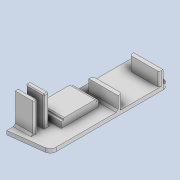
# Autodesk Inventor part: ploh
Saved by Autodesk Inventor 2020 (Build 240168000, 168)
## iProperties
Created: 2022-02-12
Part Number: ploh
Material: Типовые
Document SubType Name: Modeling
Designer: korra
Density: 1 g/cm^3
Appearance: По умолчанию
Author: korra
Autodesk Inventor part; units mm, degrees
ref_plane "YZ Plane" through (0, 0, 0) normal (1, 0, 0) x (0, 1, 0)
ref_plane "XZ Plane" through (0, 0, 0) normal (0, 1, 0) x (-1, 0, 0)
ref_plane "XY Plane" through (0, 0, 0) normal (0, 0, 1) x (1, 0, 0)
sketch "Эскиз1" plane through (0, 0, 0) normal (0, 1, 0) x (-1, 0, 0)
  line L0 (-5, 11.7093) -> (-5, -48.2907)
  line L1 (15, 10.2093) -> (15, -46.7907)
  line L2 (15, 10.2093) -> (15, 14.2093)
  line L3 (15, -46.7907) -> (15, -50.7907)
  line L4 (15, 14.2093) -> (-5, 11.7093)
  line L5 (15, -50.7907) -> (-5, -48.2907)
  point P0 (0, 0)
  dimension "d0" = 60
  dimension "d3" = 20
  dimension "d4" = 4
  dimension "d5" = 4
  constraints: 12 end point, 4 vertical
  measures "d0" distance of L0.start L0.end
  measures "d3" distance between parallel lines of L0 L1
  measures "d4" distance of L1.start L2.end
  measures "d5" distance of L1.end L3.end
extrude "Выдавливание1" add sketch "Эскиз1" along normal blind 2
fillet "Сопряжение1" radius 3 2 edges at (5, 1, -48.2907) (5, 1, 11.7093)
sketch "Эскиз3" plane through (0, 2, 0) normal (0, 1, 0) x (1, 0, 0)
  arc A0 (5, 45.6424) -> (2.3721, 48.6192) centre (2, 45.6424) ccw projected
  line L0 (5, 45.6424) -> (-10, 45.6424)
  line L1 (-10, 45.6424) -> (-10, 43.6424)
  line L2 (-10, 43.6424) -> (5, 43.6424)
  line L3 (5, 43.6424) -> (5, 45.6424)
  line L4 (5, -9.0609) -> (5, 45.6424) projected
  line L5 (5, 24.6424) -> (-10, 24.6424)
  line L6 (-10, 24.6424) -> (-10, 22.6424)
  line L7 (-10, 22.6424) -> (5, 22.6424)
  line L8 (5, 22.6424) -> (5, 24.6424)
  point P0 (0, 0)
  dimension "d21" = 15
  dimension "d22" = 2
  dimension "d23" = 2
  dimension "d24" = 19
  constraints: 16 end point, 4 parallel, 2 horizontal, 2 perpendicular, 1 point on line
  measures "d21" distance of L2.end L1.end
  measures "d22" distance of L0.end L1.end
  measures "d23" distance of L5.end L6.end
  measures "d24" distance between parallel lines of L2 L5
extrude "Выдавливание2" add sketch "Эскиз3" along normal blind 7
fillet "Сопряжение2" radius 1 4 edges at (5, 5.5, -43.6424) (5, 5.5, -24.6424) (-10, 5.5, -43.6424) (-10, 5.5, -24.6424)
chamfer "Фаска1" distance 1 angle 45 1 edges at (-2.5, 2, -45.6424)
sketch "Эскиз4" plane through (0, 2, 0) normal (0, 1, 0) x (1, 0, 0)
  line L0 (5, -9.0609) -> (5, 45.6424) projected
  line L1 (5, 19.6424) -> (-15, 19.6424)
  line L2 (-15, 19.6424) -> (-15, 0.5424)
  line L3 (-15, 0.5424) -> (5, 0.5424)
  line L4 (5, 0.5424) -> (5, 19.6424)
  line L5 (-9, 43.6424) -> (4, 43.6424) projected
  point P0 (0, 0)
  point P1 (5, 0.5424)
  dimension "d31" = 20
  dimension "d32" = 19.1
  dimension "d33" = 24
  constraints: 8 end point, 2 parallel, 1 horizontal, 1 perpendicular, 1 point on line
  measures "d31" distance of L3.end L2.end
  measures "d32" distance of L1.end L2.end
  measures "d33" distance between parallel lines of L5 L1
extrude "Выдавливание3" add sketch "Эскиз4" along normal blind 4
sketch "Эскиз5" plane through (0, 6, 0) normal (0, 1, 0) x (1, 0, 0)
  line L0 (-15, 0.5424) -> (5, 0.5424) projected
  line L1 (-15, 19.6424) -> (5, 19.6424) projected
  line L2 (5, 0.5424) -> (-2, 0.5424)
  line L3 (-2, 0.5424) -> (-2, 19.6424)
  line L4 (-2, 19.6424) -> (5, 19.6424)
  line L5 (5, 19.6424) -> (5, 0.5424)
  point P0 (0, 0)
  point P1 (5, 19.6424)
  dimension "d36" = 7
  constraints: 8 end point, 2 parallel, 1 horizontal, 1 perpendicular, 1 point on line
  measures "d36" distance of L3.end L4.end
extrude "Выдавливание4" cut sketch "Эскиз5" against normal blind 4
sketch "Эскиз6" plane through (0, 6, 0) normal (0, 1, 0) x (1, 0, 0)
  line L0 (-15, 50.7907) -> (-15, -14.2093) projected
  line L1 (-15, 0.5424) -> (-2, 0.5424) projected
  line L2 (-15, 1.7424) -> (-2, 1.7424)
  line L3 (-2, 1.7424) -> (-2, 0.5424)
  line L4 (-2, 0.5424) -> (-15, 0.5424)
  line L5 (-15, 0.5424) -> (-15, 1.7424)
  line L6 (-2, 0.5424) -> (-2, 19.6424) projected
  line L7 (-2, 19.6424) -> (-15, 19.6424)
  line L8 (-15, 19.6424) -> (-15, 18.4424)
  line L9 (-15, 18.4424) -> (-2, 18.4424)
  line L10 (-2, 18.4424) -> (-2, 19.6424)
  point P0 (0, 0)
  point P1 (-2, 18.4424)
  point P2 (-15, 19.6424)
  dimension "d39" = 1.2
  dimension "d40" = 1.2
  constraints: 16 end point, 4 parallel, 2 horizontal, 2 perpendicular, 2 point on line
  measures "d39" distance between parallel lines of L7 L9
  measures "d40" distance between parallel lines of L1 L2
extrude "Выдавливание5" cut sketch "Эскиз6" against normal blind 1 contours L7 L6 L9 L0 | L2 L3 L1 L0
fillet "Сопряжение3" radius 0.5 2 edges at (-8.5, 6, -1.7424) (-8.5, 6, -18.4424)
sketch "Эскиз7" plane through (0, 2, 0) normal (0, 1, 0) x (1, 0, 0)
  line L0 (-15, -9.8754) -> (-6, -9.8754)
  line L1 (-6, -9.8754) -> (-6, -7.8754)
  line L2 (-6, -7.8754) -> (-15, -7.8754)
  line L3 (-15, -7.8754) -> (-15, -9.8754)
  line L4 (-15, 0.5424) -> (-15, -14.2093) projected
  line L5 (-6, -2.2754) -> (-15, -2.2754)
  line L6 (-15, -2.2754) -> (-15, -4.2754)
  line L7 (-15, -4.2754) -> (-6, -4.2754)
  line L8 (-6, -4.2754) -> (-6, -2.2754)
  point P0 (0, 0)
  dimension "d44" = 2
  dimension "d45" = 0
  dimension "d46" = 9
  dimension "d47" = 2
  dimension "d48" = 3.6
  constraints: 16 end point, 4 parallel, 2 horizontal, 2 perpendicular, 1 point on line
  measures "d44" distance of L0.end L1.end
  measures "d45" distance between parallel lines of L4 L3
  measures "d46" distance of L1.end L2.end
  measures "d47" distance of L7.end L5.start
  measures "d48" distance between parallel lines of L2 L7
extrude "Выдавливание6" add sketch "Эскиз7" along normal blind 15.3
fillet "Сопряжение4" radius 0.5 8 edges at (-6, 17.3, 3.2754) (-10.5, 17.3, 4.2754) (-10.5, 17.3, 7.8754) (-6, 17.3, 8.8754) (-6, 9.65, 4.2754) (-6, 9.65, 7.8754) (-15, 9.65, 4.2754) (-15, 9.65, 7.8754)
chamfer "Фаска2" distance 1 angle 45 3 edges at (-10.5, 2, 9.8754) (-10.5, 2, 2.2754) (-2.5, 2, -22.6424)
